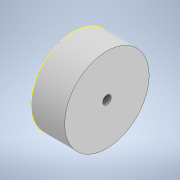
# Autodesk Inventor part: вшакькьькьк
Saved by Autodesk Inventor 2020 (Build 240168000, 168)
## iProperties
Created: 2022-04-28
Part Number: вшакькьькьк
Material: Типовые
Document SubType Name: Modeling
Designer: robokvantum
Density: 1 g/cm^3
Appearance: По умолчанию
Author: robokvantum
Autodesk Inventor part; units mm, degrees
ref_plane "YZ Plane" through (0, 0, 0) normal (1, 0, 0) x (0, 1, 0)
ref_plane "XZ Plane" through (0, 0, 0) normal (0, 1, 0) x (-1, 0, 0)
ref_plane "XY Plane" through (0, 0, 0) normal (0, 0, 1) x (1, 0, 0)
sketch "Эскиз1" plane through (0, 0, 0) normal (1, 0, 0) x (0, 1, 0)
  circle A0 centre (0, 0) radius 5
  circle A1 centre (0, 0) radius 50
  dimension "d2" = 10
  dimension "d3" = 100
  constraints: 2 centre point, 2 coincident
  measures "d2" diameter of A0
  measures "d3" diameter of A1
extrude "Выдавливание1" add sketch "Эскиз1" along normal blind 40
sketch "Эскиз2" plane through (0, 0, 0) normal (-1, 0, 0) x (0, 0, 1)
  circle A0 centre (0, 0) radius 34.3349
  circle A1 centre (0, 0) radius 50 projected
  circle A2 centre (0, 0) radius 5 projected
  circle A3 centre (0, 28.7128) radius 4.1781
  circle A4 centre (24.4962, 0) radius 4.2688
  circle A5 centre (0, -24.0946) radius 4.726
  circle A6 centre (-24.0946, 0) radius 4.2877
  circle A7 centre (-20.89, -2.8486) radius 0.1294
  constraints: 5 centre point, 1 coincident, 3 other
